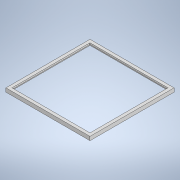
# Autodesk Inventor part: top_frame
Saved by Autodesk Inventor 2020.2 (Build 242310000, 310)
## iProperties
Created: 2021-09-14
Part Number: top_frame
Material: Generic
Document SubType Name: Modeling
Designer: Tarsoly
Density: 1 g/cm^3
Appearance: Default
Author: Tarsoly
Autodesk Inventor part; units mm, degrees
ref_plane "YZ Plane" through (0, 0, 0) normal (1, 0, 0) x (0, 1, 0)
ref_plane "XZ Plane" through (0, 0, 0) normal (0, 1, 0) x (-1, 0, 0)
ref_plane "XY Plane" through (0, 0, 0) normal (0, 0, 1) x (1, 0, 0)
sketch "Sketch1" plane through (0, 0, 0) normal (0, 1, 0) x (-1, 0, 0)
  line L0 (54.002, 54.002) -> (-54.002, 54.002) construction
  line L1 (-54.002, 54.002) -> (-54.002, -54.002) construction
  line L2 (-54.002, -54.002) -> (54.002, -54.002) construction
  line L3 (54.002, -54.002) -> (54.002, 54.002) construction
  line L4 (54.002, 54.002) -> (-54.002, -54.002) construction
  line L5 (-54.002, 54.002) -> (54.002, -54.002) construction
  line L6 (54.102, 54.102) -> (-54.102, 54.102)
  line L7 (-54.102, 54.102) -> (-54.102, -54.102)
  line L8 (-54.102, -54.102) -> (54.102, -54.102)
  line L9 (54.102, -54.102) -> (54.102, 54.102)
  line L10 (56.102, 56.102) -> (-56.102, 56.102)
  line L11 (-56.102, 56.102) -> (-56.102, -56.102)
  line L12 (-56.102, -56.102) -> (56.102, -56.102)
  line L13 (56.102, -56.102) -> (56.102, 56.102)
  line L14 (52.102, 52.102) -> (-52.102, 52.102)
  line L15 (-52.102, 52.102) -> (-52.102, -52.102)
  line L16 (-52.102, -52.102) -> (52.102, -52.102)
  line L17 (52.102, -52.102) -> (52.102, 52.102)
  point P0 (0, 0)
  dimension "d0" = 108.004
  dimension "d9" = 0.1
  dimension "d10" = 2
  dimension "d11" = 2
  constraints: 36 end point, 8 parallel, 5 perpendicular, 2 midpoint, 1 horizontal, 9 other
  measures "d0" distance of L2.end L1.end
  measures "d9" distance between parallel lines of L3 L9
  measures "d10" distance between parallel lines of L13 L9
  measures "d11" distance between parallel lines of L17 L9
extrude "Extrusion1" add sketch "Sketch1" along normal blind 2 contours L9 L8 L7 L6 | L13 L12 L11 L10
sketch "Sketch2" plane through (0, 0, 0) normal (0, -1, 0) x (1, 0, 0)
  line L0 (56.102, 56.102) -> (56.102, -56.102) projected
  line L1 (-56.102, 56.102) -> (56.102, 56.102) projected
  line L2 (-56.102, -56.102) -> (-56.102, 56.102) projected
  line L3 (56.102, -56.102) -> (-56.102, -56.102) projected
  line L4 (56.102, 56.102) -> (56.102, -56.102) projected
  line L5 (-52.102, -52.102) -> (52.102, -52.102) projected
  line L6 (-52.102, 52.102) -> (-52.102, -52.102) projected
  line L7 (52.102, 52.102) -> (-52.102, 52.102) projected
  line L8 (52.102, -52.102) -> (52.102, 52.102) projected
  line L9 (54.102, 54.102) -> (-54.102, 54.102)
  line L10 (-54.102, 54.102) -> (-54.102, -54.102)
  line L11 (-54.102, -54.102) -> (54.102, -54.102)
  line L12 (54.102, -54.102) -> (54.102, 54.102)
  point P0 (0, 0)
  dimension "d12" = 2
  constraints: 8 end point, 3 other
  measures "d12" distance between parallel lines of L7 L9
extrude "Extrusion2" add sketch "Sketch2" along normal blind 3 contours L0 L3 L2 L1
body "Solid1"
